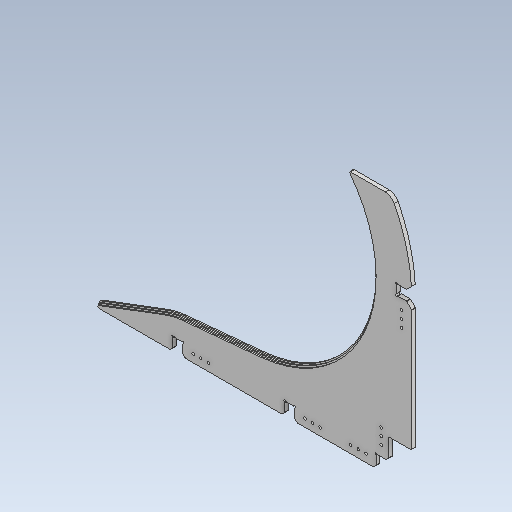
# Autodesk Inventor part: Ball_IndexerC
Saved by Autodesk Inventor 2020 (Build 240168000, 168)
## iProperties
Created: 2020-01-26
Part Number: Ball_IndexerC
Material: Generic
Document SubType Name: Modeling
Designer: srini
Density: 1 g/cm^3
Appearance: Default
Author: srini
Autodesk Inventor part; units mm, degrees
ref_plane "YZ Plane" through (0, 0, 0) normal (1, 0, 0) x (0, 1, 0)
ref_plane "XZ Plane" through (0, 0, 0) normal (0, 1, 0) x (-1, 0, 0)
ref_plane "XY Plane" through (0, 0, 0) normal (0, 0, 1) x (1, 0, 0)
sketch "Sketch1" plane through (0, 0, 0) normal (0, 0, 1) x (1, 0, 0)
  arc A0 (240.9656, 196.85) -> (28.7998, -309.8143) centre (0, 0) ccw
  line L0 (-190.5, -381) -> (-165.1, -381)
  line L1 (-165.1, -381) -> (-165.1, -406.4)
  line L2 (-165.1, -406.4) -> (-190.5, -406.4)
  line L3 (-190.5, -406.4) -> (-190.5, -381)
  line L4 (-190.5, -381) -> (-165.1, -406.4) construction
  line L5 (-165.1, -381) -> (-190.5, -406.4) construction
  line L6 (88.9, -381) -> (114.3, -381)
  line L7 (114.3, -381) -> (114.3, -406.4)
  line L8 (114.3, -406.4) -> (88.9, -406.4)
  line L9 (88.9, -406.4) -> (88.9, -381)
  line L10 (88.9, -381) -> (114.3, -406.4) construction
  line L11 (114.3, -381) -> (88.9, -406.4) construction
  line L12 (317.5, -381) -> (342.9, -381)
  line L13 (342.9, -381) -> (342.9, -406.4)
  line L14 (342.9, -406.4) -> (317.5, -406.4)
  line L15 (317.5, -406.4) -> (317.5, -381)
  line L16 (317.5, -381) -> (342.9, -406.4) construction
  line L17 (342.9, -381) -> (317.5, -406.4) construction
  circle A1 centre (-374.65, -406.4) radius 6.35
  line L18 (-190.5, -330.2) -> (28.7998, -309.8143)
  line L19 (-374.65, -412.75) -> (-196.85, -412.75)
  line L20 (349.25, -374.65) -> (349.25, -328.676)
  line L21 (349.25, -328.676) -> (406.4, -328.676)
  line L22 (406.4, -328.676) -> (406.4, -25.4)
  arc A2 (406.4, 0) -> (405.6516, 24.6516) centre (0, 0) ccw
  line L23 (355.5433, 196.85) -> (240.9656, 196.85)
  arc A3 (28.7998, -309.8143) -> (240.9656, 196.85) centre (0, 0) ccw
  line L24 (-190.5, -406.4) -> (-196.85, -412.75)
  line L25 (-165.1, -406.4) -> (-158.75, -412.75)
  line L26 (88.9, -406.4) -> (82.55, -412.75)
  line L27 (114.3, -406.4) -> (120.65, -412.75)
  line L28 (317.5, -406.4) -> (311.15, -412.75)
  line L29 (-196.85, -412.75) -> (-158.75, -412.75)
  line L30 (-158.75, -412.75) -> (82.55, -412.75)
  line L31 (82.55, -412.75) -> (120.65, -412.75)
  line L32 (120.65, -412.75) -> (311.15, -412.75)
  line L33 (342.9, -381) -> (349.25, -374.65)
  line L34 (393.7, -12.7) -> (368.3, -12.7)
  line L35 (368.3, -12.7) -> (368.3, 12.7)
  line L36 (368.3, 12.7) -> (393.7, 12.7)
  line L37 (393.7, 12.7) -> (393.7, -12.7)
  line L38 (393.7, -12.7) -> (368.3, 12.7) construction
  line L39 (368.3, -12.7) -> (393.7, 12.7) construction
  line L40 (393.7, -12.7) -> (406.4, -25.4)
  line L41 (393.7, 12.7) -> (405.6516, 24.6516)
  line L42 (406.4, -25.4) -> (406.4, 0)
  arc A4 (405.6516, 24.6516) -> (355.5433, 196.85) centre (0, 0) ccw
  line L43 (-190.5, -330.2) -> (-376.8897, -400.4581)
  point P0 (-177.8, -393.7)
  point P1 (101.6, -393.7)
  point P2 (330.2, -393.7)
  point P3 (-177.8, -393.7)
  point P4 (101.6, -393.7)
  point P5 (101.6, -393.7)
  point P6 (330.2, -393.7)
  point P7 (381, 0)
  point P8 (381, 0)
  dimension "d0" = 622.3
  dimension "d1" = 25.4
  dimension "d2" = 279.4
  dimension "d3" = 228.6
  dimension "d4" = 190.5
  dimension "d5" = 406.4
  dimension "d6" = 12.7
  dimension "d7" = 184.15
  dimension "d8" = 12.7
  dimension "d9" = 596.9
  dimension "d10" = 77.724
  dimension "d11" = 609.6
  dimension "d12" = 406.4
  dimension "d13" = 25.4
  dimension "d16" = 0
  dimension "d17" = 50.8
  constraints: 88 end point, 17 perpendicular, 13 midpoint, 11 point on line, 11 tangent, 10 horizontal, 10 point on circle, 9 parallel, 8 equal length, 5 centre point, 4 collinear, 3 horizontal alignment, 1 coincident, 1 concentric, 1 vertical
  measures "d0" diameter of A0
  measures "d1" distance of L0.start L0.end
  measures "d2" distance between parallel lines of L9 L3
  measures "d3" distance between parallel lines of L15 L9
  measures "d4" distance from line of L3 point (0, 0)
  measures "d5" distance from line of L2 point (0, 0)
  measures "d6" diameter of A1
  measures "d7" distance from line of A1.centre L3
  measures "d8" vertical distance of A1.centre point (-177.8, -393.7)
  measures "d9" distance between parallel lines of L3 L22
  measures "d10" distance between parallel lines of L21 L14
  measures "d11" distance between parallel lines of L32 L23
  measures "d12" radius of A2
  measures "d13" distance between parallel lines of L13 L35
  measures "d16" horizontal distance of L18.start L0.start
  measures "d17" distance from line of L18.start L0
extrude "Extrusion1" add sketch "Sketch1" along normal blind 9.525 contours L23 A4 L41 L36 L35 L34 L40 L22 L21 L20 L33 L12 L15 L28 L32 L27 L7 L6 L9 L26 L30 L25 L1 L0 L3 L24 L19 A1 L43 L18 A3 | A1
fillet "Fillet1" radius 177.8 1 edges at (-190.5, -330.2, 4.7625)
fillet "Fillet1" radius 25.4 1 edges at (355.5433, 196.85, 4.7625)
fillet "Fillet1" radius 6.35 1 edges at (240.9656, 196.85, 4.7625)
fillet "Fillet1" radius 1.5875 18 edges at (-190.5, -406.4, 4.7625) (-165.1, -406.4, 4.7625) (-158.75, -412.75, 4.7625) (-196.85, -412.75, 4.7625) (82.55, -412.75, 4.7625) (88.9, -406.4, 4.7625) (114.3, -406.4, 4.7625) (120.65, -412.75, 4.7625) (311.15, -412.75, 4.7625) (317.5, -406.4, 4.7625) (342.9, -381, 4.7625) (349.25, -374.65, 4.7625) (406.4, -328.676, 4.7625) (349.25, -328.676, 4.7625) (406.4, -25.4, 4.7625) (393.7, -12.7, 4.7625) (393.7, 12.7, 4.7625) (405.6516, 24.6516, 4.7625)
sketch "Sketch2" plane through (0, 0, 9.525) normal (0, 0, 1) x (1, 0, 0)
  circle A0 centre (-139.7, -393.7) radius 3.3734
  circle A1 centre (139.7, -393.7) radius 3.3734
  circle A2 centre (254, -393.7) radius 3.3734
  line L0 (-165.1, -381) -> (-165.1, -405.7424) projected
  line L1 (-190.5, -381) -> (-165.1, -381) projected
  line L2 (114.3, -381) -> (114.3, -405.7424) projected
  line L3 (317.5, -405.7424) -> (317.5, -381) projected
  circle A3 centre (-120.65, -393.7) radius 3.3734
  circle A4 centre (158.75, -393.7) radius 3.3734
  circle A5 centre (273.05, -393.7) radius 3.3734
  circle A6 centre (-101.6, -393.7) radius 3.3734
  circle A7 centre (177.8, -393.7) radius 3.3734
  circle A8 centre (292.1, -393.7) radius 3.3734
  circle A9 centre (381, -38.1) radius 3.3734
  circle A10 centre (330.2, -317.5) radius 3.3734
  line L4 (393.0424, -12.7) -> (368.3, -12.7) projected
  line L5 (368.3, -12.7) -> (368.3, 12.7) projected
  line L6 (317.5, -381) -> (342.2424, -381) projected
  circle A11 centre (381, -57.15) radius 3.3734
  circle A12 centre (330.2, -336.55) radius 3.3734
  circle A13 centre (381, -76.2) radius 3.3734
  circle A14 centre (330.2, -355.6) radius 3.3734
  line L7 (-190.5, -405.7424) -> (-190.5, -381) projected
  circle A15 centre (-190.5, -381) radius 2.2225
  line L8 (-190.5, -381) -> (-165.1, -381) projected
  circle A16 centre (-165.1, -381) radius 2.2225
  line L9 (88.9, -405.7424) -> (88.9, -381) projected
  circle A17 centre (88.9, -381) radius 2.2225
  line L10 (88.9, -381) -> (114.3, -381) projected
  circle A18 centre (114.3, -381) radius 2.2225
  line L11 (317.5, -381) -> (342.2424, -381) projected
  circle A19 centre (317.5, -381) radius 2.2225
  line L12 (393.0424, -12.7) -> (368.3, -12.7) projected
  circle A20 centre (368.3, -12.7) radius 2.2225
  line L13 (368.3, -12.7) -> (368.3, 12.7) projected
  circle A21 centre (368.3, 12.7) radius 2.2225
  point P0 (0, 0)
  dimension "d22" = 6.7469
  dimension "d23" = 25.4
  dimension "d24" = 12.7
  dimension "d25" = 25.4
  dimension "d26" = 63.5
  dimension "d29" = 19.05
  dimension "d34" = 25.4
  dimension "d35" = 12.7
  dimension "d36" = 12.7
  dimension "d37" = 63.5
  dimension "d40" = 19.05
  dimension "d45" = 4.445
  constraints: 22 centre point, 10 equal radius, 6 coincident, 2 horizontal alignment, 1 horizontal, 1 vertical, 20 other
  measures "d22" diameter of A0
  measures "d23" distance from line of A0.centre L0
  measures "d24" distance from line of A0.centre L1
  measures "d25" distance from line of A1.centre L2
  measures "d26" distance from line of A2.centre L3
  measures "d29" distance of A0.centre A3.centre
  measures "d34" distance from line of A9.centre L4
  measures "d35" distance from line of A9.centre L5
  measures "d36" distance from line of A10.centre L3
  measures "d37" distance from line of A10.centre L6
  measures "d40" distance of A9.centre A11.centre
  measures "d45" diameter of A15
extrude "Extrusion2" cut sketch "Sketch2" against normal through all
fillet "Fillet2" radius 1.5875 14 edges at (-190.5, -383.2225, 4.7625) (-188.2775, -381, 4.7625) (-167.3225, -381, 4.7625) (-165.1, -383.2225, 4.7625) (88.9, -383.2225, 4.7625) (91.1225, -381, 4.7625) (112.0775, -381, 4.7625) (114.3, -383.2225, 4.7625) (317.5, -383.2225, 4.7625) (319.7225, -381, 4.7625) (368.3, -10.4775, 4.7625) (370.5225, -12.7, 4.7625) (368.3, 10.4775, 4.7625) (370.5225, 12.7, 4.7625)
sketch "Sketch3" plane through (0, 0, 9.525) normal (0, 0, 1) x (1, 0, 0)
  line L0 (-212.9098, -338.6472) -> (-376.8897, -400.4581) projected
  arc A0 (-166.6539, -327.9833) -> (-212.9098, -338.6472) centre (-150.1968, -505.02) ccw projected
  line L1 (28.7998, -309.8143) -> (-166.6539, -327.9833) projected
  arc A1 (28.7998, -309.8143) -> (248.92, 186.69) centre (0, 0) ccw projected
  arc A2 (29.0936, -312.9757) -> (250.5186, 189.8437) centre (0, 0) ccw
  line L2 (29.0936, -312.9757) -> (-166.36, -331.1447)
  arc A3 (-166.36, -331.1447) -> (-211.7899, -341.6181) centre (-150.1968, -505.02) ccw
  line L3 (-211.7899, -341.6181) -> (-376.3112, -403.6331)
  arc A4 (-376.8897, -400.4581) -> (-374.65, -412.75) centre (-374.65, -406.4) ccw projected
  arc A5 (254, 196.85) -> (248.92, 186.69) centre (254, 190.5) ccw projected
  arc A6 (254, 196.85) -> (248.92, 186.69) centre (254, 190.5) ccw projected
  arc A7 (254, 196.85) -> (250.5186, 189.8437) centre (254, 192.4819) ccw
  line L4 (340.2439, 196.85) -> (254, 196.85) projected
  arc A8 (-376.8897, -400.4581) -> (-374.65, -412.75) centre (-374.65, -406.4) ccw projected
  arc A9 (-376.3112, -403.6331) -> (-374.65, -412.75) centre (-374.65, -408.0402) ccw
  line L5 (-374.65, -412.75) -> (-197.5076, -412.75) projected
  dimension "d49" = 3.175
  constraints: 8 point on circle, 4 centre point, 4 end point, 4 tangent, 3 other
  measures "d49" radial gap between concentric circles of A1 A2
extrude "Extrusion3" cut sketch "Sketch3" against normal blind 6.35
sketch "Sketch4" plane through (0, 0, 9.525) normal (0, 0, 1) x (1, 0, 0)
  arc A0 (29.0936, -312.9757) -> (250.5186, 189.8437) centre (0, 0) ccw projected
  line L0 (29.0936, -312.9757) -> (-166.36, -331.1447) projected
  arc A1 (-166.36, -331.1447) -> (-211.7899, -341.6181) centre (-150.1968, -505.02) ccw projected
  line L1 (-211.7899, -341.6181) -> (-376.3112, -403.6331) projected
  line L2 (-375.7327, -406.8081) -> (-210.67, -344.5891)
  arc A2 (-166.0661, -334.306) -> (-210.67, -344.5891) centre (-150.1968, -505.02) ccw
  line L3 (-166.0661, -334.306) -> (29.3875, -316.137)
  arc A3 (29.3875, -316.137) -> (252.1015, 193.0055) centre (0, 0) ccw
  line L4 (-374.65, -412.75) -> (-197.5076, -412.75) projected
  arc A4 (-375.7327, -406.8081) -> (-374.65, -412.75) centre (-374.65, -409.6804) ccw
  arc A5 (-376.3112, -403.6331) -> (-374.65, -412.75) centre (-374.65, -408.0402) ccw projected
  arc A6 (254, 196.85) -> (248.92, 186.69) centre (254, 190.5) ccw projected
  arc A7 (254, 196.85) -> (252.1015, 193.0055) centre (254, 194.459) ccw
  line L5 (340.2439, 196.85) -> (254, 196.85) projected
  arc A8 (254, 196.85) -> (250.5186, 189.8437) centre (254, 192.4819) ccw projected
  dimension "d52" = 3.175
  constraints: 8 point on circle, 4 centre point, 4 end point, 4 tangent, 3 other
  measures "d52" distance between parallel lines of L3 L0
extrude "Extrusion4" cut sketch "Sketch4" against normal blind 3.175
equation "\"d50\" = 0.666667 * d14"
equation "\"d53\" = 0.333333 * d14"
equation "\"d14\" = 9.525"
body "Solid1"
